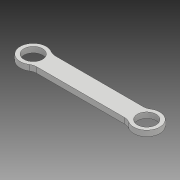
# Autodesk Inventor part: tendon
Saved by Autodesk Inventor 2017 SP1 (Build 210196100, 196)
## iProperties
Created: 2017-06-23
Part Number: tendon
Material: Generic
Document SubType Name: Modeling
Designer: Tomasz
Density: 1 g/cm^3
Appearance: Default
Author: Tomasz
Autodesk Inventor part; units mm, degrees
ref_plane "YZ Plane" through (0, 0, 0) normal (1, 0, 0) x (0, 1, 0)
ref_plane "XZ Plane" through (0, 0, 0) normal (0, 1, 0) x (-1, 0, 0)
ref_plane "XY Plane" through (0, 0, 0) normal (0, 0, 1) x (1, 0, 0)
sketch "Sketch1" plane through (0, 0, 0) normal (0, 0, 1) x (1, 0, 0)
  line L0 (-15.2, 0) -> (15.2, 0) construction
  arc A0 (-12.7505, 2.5) -> (-12.7505, -2.5) centre (-15.2, 0) ccw
  arc A1 (12.7505, -2.5) -> (12.7505, 2.5) centre (15.2, 0) ccw
  line L1 (-12.7505, 2.5) -> (12.7505, 2.5)
  line L2 (12.7505, -2.5) -> (-12.7505, -2.5)
  point P0 (0, 0)
  point P1 (0, 0)
  dimension "d0" = 3.5
  dimension "d1" = 30.4
  dimension "d26" = 3.5
  dimension "d27" = 5
  constraints: 8 end point, 4 point on circle, 2 centre point, 2 coincident, 2 horizontal, 2 vertical alignment, 1 midpoint
  measures "d0" radius of A0
  measures "d1" distance of L0.end L0.start
  measures "d26" radius of A1
  measures "d27" distance of L2.end L1.start
extrude "Extrusion1" add sketch "Sketch1" along normal blind 1.5
hole "Hole1" at (-15.2, 0, 1.5) direction (0, 0, -1) diameter 5 end through all
hole "Hole2" at (15.2, 0, 1.5) direction (0, 0, -1) diameter 5 end through all
fillet "Fillet1" radius 3 4 edges at (-12.7505, -2.5, 0.75) (12.7505, -2.5, 0.75) (12.7505, 2.5, 0.75) (-12.7505, 2.5, 0.75)
body "Solid1"
